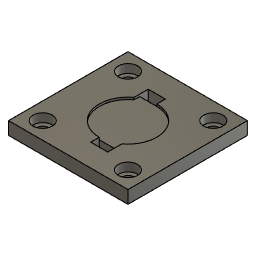
Démareur v3 (Autodesk Fusion 360 design; units mm, degrees)
Autodesk Fusion 360 part; units mm, degrees
note: some values were not read from the file. Set by a fixed rule: which sketch regions a step uses.
sketch "Sketch1" plane through (0, 0, 0) normal (0, 1, 0) x (1, 0, 0)
  line L0 (-14, 14) -> (14, 14)
  line L1 (14, 14) -> (14, -14)
  line L2 (14, -14) -> (-14, -14)
  line L3 (-14, -14) -> (-14, 14)
  line L4 (-14, 14) -> (14, -14) construction
  circle A0 centre (0, 0) radius 6.75
  line L5 (-4, 8.75) -> (0, 8.75)
  line L6 (0, 8.75) -> (0, 6.75)
  line L7 (0, 6.75) -> (-4, 6.75)
  line L8 (-4, 6.75) -> (-4, 8.75)
  line L9 (0, 0) -> (0, 6.75)
  line L10 (0, 0) -> (0, -6.75)
  line L11 (0, -6.75) -> (4, -6.75)
  line L12 (4, -6.75) -> (4, -8.75)
  line L13 (4, -8.75) -> (0, -8.75)
  line L14 (0, -8.75) -> (0, -6.75)
  line L15 (10, -10) -> (-10, -10) construction
  line L16 (-10, -10) -> (-10, 10) construction
  line L17 (-10, 10) -> (10, 10) construction
  line L18 (10, 10) -> (10, -10) construction
  circle A1 centre (-10, 10) radius 1.25
  circle A2 centre (10, 10) radius 1.25
  circle A3 centre (-10, -10) radius 1.25
  circle A4 centre (10, -10) radius 1.25
  line L19 (4, -6.75) -> (4, -5.4371)
  line L20 (-4, 6.75) -> (-4, 5.4371)
  circle A5 centre (-10, -10) radius 2.25
  circle A6 centre (-10, 10) radius 2.25
  circle A7 centre (10, 10) radius 2.25
  circle A8 centre (10, -10) radius 2.25
  dimension "d1" = 28
  dimension "d2" = 28
  dimension "d3" = 13.5
  dimension "d4" = 4
  dimension "d5" = 2
  dimension "d8" = 4
  dimension "d9" = 2
  dimension "d10" = 4
  dimension "d11" = 2.5
  dimension "d12" = 2.5
  dimension "d13" = 2.5
  dimension "d14" = 2.5
  dimension "d20" = 4.5
  dimension "d21" = 4.5
  dimension "d22" = 4.5
  dimension "d23" = 4.5
  constraint horizontal L0
  constraint vertical L1
  constraint horizontal L2
  constraint vertical L3
  constraint midpoint L4 A0.centre
  constraint midpoint A0.centre L4
  constraint coincident A0.centre L9.start
  constraint horizontal L5
  constraint vertical L6
  constraint horizontal L7
  constraint vertical L8
  constraint coincident A0 L6.end
  constraint vertical L9
  constraint coincident A0 L10.end
  constraint parallel L9 L10
  constraint horizontal L11
  constraint vertical L12
  constraint horizontal L13
  constraint vertical L14
  constraint coincident L16.end L17.start
  constraint coincident L17.end L18.start
  constraint coincident L15.end L16.start
  constraint coincident L15.start L18.end
  constraint coincident A0 L19.end
  constraint perpendicular L11 L19
  constraint coincident A0 L20.end
  constraint perpendicular L7 L20
  constraint concentric A3 A5
  constraint concentric A1 A6
  constraint concentric A2 A7
  constraint concentric A4 A8
  measures "d1" distance of L0.start L0.end
  measures "d2" distance of L0.start L2.end
  measures "d3" diameter of A0
  measures "d4" distance of L5.start L5.end
  measures "d5" distance of L5.start L7.end
  measures "d8" distance of L10.end L11.end
  measures "d9" distance of L10.end L13.end
  measures "d11" diameter of A1
  measures "d12" diameter of A2
  measures "d13" diameter of A3
  measures "d14" diameter of A4
  measures "d20" diameter of A5
  measures "d21" diameter of A6
  measures "d22" diameter of A7
  measures "d23" diameter of A8
extrude "Extrude1" add sketch "Sketch1" along normal blind 3 contours L0 L1 L2 L3 | A0 L9 L10 | A0 L9 L10 | A0 L7 L20 | A0 L11 L19 | A5 | A6 | A7 | A8
extrude "Extrude2" cut sketch "Sketch1" against normal blind 0.5 from surface at 3 contours A0 L9 L10 | A0 L9 L10 | A0 L7 L20 | A0 L11 L19
extrude "Extrude3" cut sketch "Sketch1" against normal blind 2 from surface at 3 contours A2 | A5 | A6 | A7 | A8
equation "d1 = d2"
named bodies: "Demarreur"
